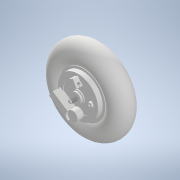
# Autodesk Inventor part: FreeBackWheel
Saved by Autodesk Inventor 2022.2 (Build 262287000, 287)
## iProperties
Created: 2022-03-30
Part Number: FreeBackWheel
Material: Generic
Document SubType Name: Modeling
Designer: Finn Oriwohl
Density: 1 g/cm^3
Appearance: Default
Author: Finn Oriwohl
Autodesk Inventor part; units mm, degrees
ref_plane "YZ Plane" through (0, 0, 0) normal (1, 0, 0) x (0, 1, 0)
ref_plane "XZ Plane" through (0, 0, 0) normal (0, 1, 0) x (-1, 0, 0)
ref_plane "XY Plane" through (0, 0, 0) normal (0, 0, 1) x (1, 0, 0)
sketch "Sketch2" plane through (0, 0, 0) normal (1, 0, 0) x (0, 1, 0)
  line L0 (17.5, 10) -> (-17.5, 10)
  line L1 (-17.5, 10) -> (-17.5, -30)
  line L2 (-17.5, -30) -> (17.5, -30)
  line L3 (17.5, -30) -> (17.5, 10)
  line L4 (17.5, 10) -> (-17.5, -30) construction
  line L5 (-17.5, 10) -> (17.5, -30) construction
  line L6 (-55, -11) -> (55, -11)
  line L7 (55, -11) -> (55, -21)
  line L8 (55, -21) -> (-55, -21)
  line L9 (-55, -21) -> (-55, -11)
  line L10 (-55, -11) -> (55, -21) construction
  line L11 (55, -11) -> (-55, -21) construction
  line L12 (46, -11) -> (46, -21)
  line L13 (-5.7139, -11) -> (24.0923, -11)
  line L14 (0, 65.6557) -> (0, -65.6557)
  circle A0 centre (73.275, 0) radius 26.725
  line L15 (0, 0) -> (82.4805, 0) construction
  line L16 (-55, 11) -> (55, 11)
  line L17 (55, 11) -> (55, 21)
  line L18 (55, 21) -> (-55, 21)
  line L19 (-55, 21) -> (-55, 11)
  line L20 (46, 11) -> (46, 21)
  line L21 (0, 31) -> (49, 31)
  line L22 (49, 31) -> (49, 21)
  line L23 (0, 38) -> (12.5, 38)
  line L24 (12.5, 38) -> (12.5, 31)
  line L25 (0, -30) -> (5, -30)
  line L26 (5, -30) -> (5, -47.5)
  line L27 (5, -47.5) -> (0, -47.5)
  line L28 (0, -47.5) -> (0, -30)
  line L29 (0, 38) -> (5, 38)
  line L30 (5, 38) -> (5, 53.8)
  line L31 (5, 53.8) -> (0, 53.8)
  line L32 (0, 53.8) -> (0, 38)
  point P0 (0, -10)
  point P1 (0, -10)
  point P2 (0, -16)
  point P3 (0, -16)
  point P4 (0, -16)
  point P5 (0, -10)
  point P6 (55, -19.5)
  point P7 (0, 16)
  point P8 (55, 19.5)
  point P9 (55, 19.5)
  point P10 (0, -30)
  point P11 (17.5, -21)
  point P12 (0, -47.5)
  point P13 (100, 0)
  dimension "d0" = 35
  dimension "d1" = 40
  dimension "d2" = 10
  dimension "d3" = 110
  dimension "d4" = 10
  dimension "d7" = 9
  dimension "d8" = 19
  dimension "d9" = 10
  dimension "d11" = 1.5
  dimension "d12" = 49
  dimension "d13" = 10
  dimension "d14" = 12.5
  dimension "d15" = 7
  dimension "d42" = 5
  dimension "d43" = 17.5
  dimension "d44" = 5
  dimension "d45" = 15.8
  dimension "d53" = 100
  constraints: 66 end point, 14 point on line, 10 midpoint, 8 horizontal, 8 parallel, 8 symmetric about line, 5 perpendicular, 3 vertical, 2 coincident, 2 point on circle, 1 centre point
  measures "d0" distance of L2.end L1.end
  measures "d1" distance of L1.end L0.end
  measures "d2" distance of point (0, -10) point (0, 0)
  measures "d3" distance of L7.end L8.end
  measures "d4" distance of L6.end L7.end
  measures "d7" distance between parallel lines of L7 L12
  measures "d8" distance between parallel lines of L2 L13
  measures "d9" distance between parallel lines of L13 L8
  measures "d11" distance of L7.end A0.start
  measures "d12" distance of L21.start L21.end
  measures "d13" distance between parallel lines of L18 L21
  measures "d14" distance of L23.start L23.end
  measures "d15" distance between parallel lines of L21 L23
  measures "d42" distance of L26.end L27.end
  measures "d43" distance of L25.end L26.end
  measures "d44" distance of L31.end L30.end
  measures "d45" distance of L30.end L29.end
  measures "d53" distance of point (0, 0) A0.end
revolve "Revolution1" add sketch "Sketch2" angle 360 about axis through (0, 0, 65.6557) along (0, 0, -1) contours L3 L6 L14 L0 | L0 L14 L16 A0 L6 L3 | L6 L12 L8 L3 | L3 L8 L14 L6 | L14 L18 L20 L16 | L3 L2 L14 L8 | L14 L21 L22 L18 | L20 L18 L17 A0 L16 | L12 L6 A0 L7 L8 | L14 L23 L24 L21 | L16 L17 A0 L7 L6 | A0 L17 L16 | L2 L26 L27 L14 | L6 L7 A0 | L14 L31 L30 L23
sketch "Sketch4" plane through (0, 0, 31) normal (0, 0, 1) x (1, 0, 0)
  circle A0 centre (32.15, 0) radius 6.15
  circle A1 centre (32.15, 0) radius 2.15
  circle A2 centre (0, 0) radius 49 projected
  circle A3 centre (0, 0) radius 49 projected
  line L0 (26, 14.6294) -> (26, -8.2066)
  circle A4 centre (0, 0) radius 36
  circle A5 centre (0, 0) radius 15
  line L1 (-8.8861, 39.8) -> (0.1206, 45)
  line L2 (0.1206, 45) -> (9.8706, 28.1125)
  line L3 (9.8706, 28.1125) -> (0.8639, 22.9125)
  line L4 (0.8639, 22.9125) -> (-8.8861, 39.8)
  line L5 (-8.8861, 39.8) -> (9.8706, 28.1125) construction
  line L6 (0.1206, 45) -> (0.8639, 22.9125) construction
  line L7 (0, 0) -> (49, 0) construction
  circle A6 centre (0.4923, -33.9563) radius 12
  line L8 (0.5569, -29.2189) -> (-43.347, -0.503)
  line L9 (-43.347, -0.503) -> (-52.105, -13.8932)
  line L10 (-52.105, -13.8932) -> (-6.0762, -43.9989)
  line L11 (-4.0111, 31.3563) -> (-50.7764, 4.3563) construction
  point P0 (0, 0)
  point P1 (0.4923, 33.9563)
  point P2 (5.5667, 35.567)
  point P3 (35.6423, 5.0622)
  point P4 (35.6423, -5.0622)
  point P5 (-6.3647, 35.4329)
  point P6 (0.4923, 33.9563)
  point P7 (-6.7865, -24.4159)
  point P8 (-48.9, 3.1289)
  point P9 (-45.4855, -18.2228)
  point P10 (-48.3238, -8.1121)
  dimension "d55" = 24
  dimension "d24" = 12.3
  dimension "d25" = 4
  dimension "d26" = 23
  dimension "d29" = 72
  dimension "d30" = 30
  dimension "d31" = 10.4
  dimension "d32" = 19.5
  dimension "d33" = 60
  dimension "d34" = 98
  dimension "d35" = 45
  dimension "d54" = 46.4246
  dimension "d56" = 16
  dimension "d57" = 54
  dimension "d62" = 55
  constraints: 24 end point, 4 centre point, 4 midpoint, 3 coincident, 3 parallel, 3 perpendicular, 2 point on line, 1 horizontal, 1 horizontal alignment, 1 symmetric about line, 1 tangent, 1 vertical, 5 other
  measures "d24" diameter of A0
  measures "d25" radial gap between concentric circles of A0 A1
  measures "d26" distance from line of L7.end L0
  measures "d29" diameter of A4
  measures "d30" diameter of A5
  measures "d31" distance of L2.end L3.end
  measures "d32" distance of L1.end L2.end
  measures "d33" angle of L0 L3
  measures "d34" diameter of A2
  measures "d35" vertical distance of A2.centre L1.end
  measures "d54" distance of A0.centre point (0.492, 33.956)
  measures "d56" distance of L8.end L9.end
  measures "d57" distance of L11.start L11.end
  measures "d62" distance from line of point (0.492, -33.956) L9
extrude "Extrusion1" add sketch "Sketch4" along normal blind 6 contours A0 A4 | A4 A0
extrude "Extrusion2" add sketch "Sketch4" along normal blind 1.5 contours A0 A4 L2 L1 L4 L8 L9 A2 L10 A6 | A6 A4 | A6 L10 A2 L9 L8 A4 picked at (0.1047, -39.1419)
extrude "Extrusion3" add sketch "Sketch4" along normal blind 2.5 contours A5
extrude "Extrusion4" add sketch "Sketch4" along normal blind 14.5 contours L2 L3 L4 A4 | A4 L4 L1 L2
sketch "Sketch3" plane through (0, 0, 38) normal (0, 0, 1) x (1, 0, 0)
  point P0 (0, 0)
  point P1 (0, 0)
  constraints: 1 coincident
hole "Hole1" [suppressed]
chamfer "Chamfer1" distance 2 angle 45 2 edges at (0, -5, 53.8) (0, -5, -47.5)
thread "Thread1" size "M10x1.5" class "6g" standard "ANSI Metric M Profile" length 14 offset 3.5
thread "Thread2" size "M10x1.5" class "6g" standard "ANSI Metric M Profile" full length
extrude "Extrusion5" add sketch "Sketch4" along normal blind 15 contours A6 A4 | A4 A6
extrude "Extrusion6" add sketch "Sketch4" along normal blind 20 contours A6 L10 A2 L9 L8 A4 | A4 L8 A6 | L10 L9 A2
sketch "Sketch5" plane through (9.8706, 28.1125, 45.5) normal (0.8660254, 0.5, 0) x (0, 0, -1)
  line L0 (13, 19.5) -> (13, 8.6077) projected
  line L1 (13, 19.5) -> (0, 19.5) projected
  line L2 (0, 0) -> (0, 19.5) projected
  line L3 (14.5, 0) -> (0, 0) projected
  line L4 (14.5, 8.6077) -> (14.5, 0) projected
  line L5 (14.5, 8.6077) -> (13, 8.6077) projected
  circle A0 centre (7.5, 5.5) radius 4
  line L6 (3.5, 17.7174) -> (3.5, 4.9566) construction
  line L7 (3.5, 9.5) -> (10.4741, 9.5) construction
  line L8 (14.5, 0) -> (0, 0) projected
  line L9 (6.5, 0) -> (6.5, 5.5)
  line L10 (8.5, 5.5) -> (8.5, 0)
  line L11 (6.5, 5.5) -> (8.5, 5.5) construction
  point P0 (45.5, -19.4108)
  point P1 (8.5, 2.75)
  point P2 (6.5, 2.75)
  point P3 (6.5, 1.627)
  point P4 (6.5, 0)
  point P5 (8.5, 1.627)
  dimension "d63" = 8
  dimension "d64" = 3.5
  dimension "d65" = 10
  dimension "d66" = 2
  constraints: 10 end point, 3 midpoint, 3 point on line, 2 perpendicular, 2 tangent, 1 centre point, 1 coincident, 1 horizontal, 1 parallel, 1 vertical
  measures "d63" diameter of A0
  measures "d64" distance between parallel lines of L2 L6
  measures "d65" distance between parallel lines of L1 L7
  measures "d66" distance of point (8.5, 2.75) point (6.5, 2.75)
extrude "Extrusion7" cut sketch "Sketch5" against normal up to surface (10.4 mm away) contours L9 A0 L10 L3 | A0
extrude "Extrusion8" cut sketch "Sketch5" against normal through all contours L9 A0 L10 L3
equation "\"d42\" = d44"
body "Solid1"
